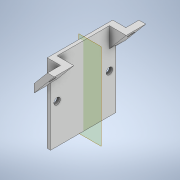
# Autodesk Inventor part: conecter bracet cover plate
Saved by Autodesk Inventor 2021 (Build 250183000, 183)
## iProperties
Created: 2022-03-10
Part Number: conecter bracet cover plate
Material: Generic
Document SubType Name: Modeling
Designer: jasmi
Density: 1 g/cm^3
Appearance: Default
Author: jasmi
Autodesk Inventor part; units mm, degrees
ref_plane "YZ Plane" through (0, 0, 0) normal (1, 0, 0) x (0, 1, 0)
ref_plane "XZ Plane" through (0, 0, 0) normal (0, 1, 0) x (-1, 0, 0)
ref_plane "XY Plane" through (0, 0, 0) normal (0, 0, 1) x (1, 0, 0)
sketch "Sketch1" plane through (0, 0, 0) normal (1, 0, 0) x (0, 1, 0)
  line L0 (76.2, 63.5) -> (0, 63.5)
  line L1 (0, 63.5) -> (0, 0)
  line L2 (0, 0) -> (76.2, 0)
  line L3 (76.2, 0) -> (76.2, 63.5)
  dimension "d0" = 76.2
  dimension "d1" = 63.5
  constraints: 8 end point, 2 parallel, 1 horizontal, 1 perpendicular
  measures "d0" distance of L1.end L2.end
  measures "d1" distance between parallel lines of L0 L2
extrude "Extrusion1" add sketch "Sketch1" along normal blind 3.175
sketch "Sketch2" plane through (3.175, 0, 0) normal (1, 0, 0) x (0, 0, -1)
  line L0 (-63.5, 76.2) -> (-63.5, 0) projected
  line L1 (0, 0) -> (0, 76.2) projected
  line L2 (0, 76.2) -> (-63.5, 76.2) projected
  point P0 (-57.15, 38.1)
  point P1 (-6.35, 38.1)
  dimension "d11" = 6.35
  dimension "d12" = 6.35
  dimension "d13" = 38.1
  dimension "d14" = 38.1
  measures "d11" distance from line of point (-57.15, 38.1) L0
  measures "d12" distance from line of point (-6.35, 38.1) L1
  measures "d13" distance from line of point (-6.35, 38.1) L2
  measures "d14" distance from line of point (-57.15, 38.1) L2
hole "Hole1" at (3.175, 38.1, 57.15) at (3.175, 38.1, 6.35) direction (-1, 0, 0) diameter 6.35 end through all
sketch "Sketch3" plane through (0, 0, 0) normal (0, 0, -1) x (-1, 0, 0)
  line L0 (-19.5018, 76.2) -> (-3.175, 56.7425)
  line L1 (-3.175, 56.7425) -> (-3.175, 76.2)
  line L2 (-3.175, 0) -> (-3.175, 76.2) projected
  line L3 (-3.175, 76.2) -> (-19.5018, 76.2)
  line L4 (0, 76.2) -> (-3.175, 76.2) projected
  point P0 (0, 0)
  dimension "d15" = 40
  dimension "d18" = 25.4
  constraints: 6 end point, 1 collinear, 1 horizontal, 1 point on line
  measures "d15" angle of L1 L0
  measures "d18" distance of L0.start L0.end
extrude "Extrusion2" add sketch "Sketch3" against normal blind 6.35
sketch "Sketch4" plane through (0, 0, 0) normal (0, 0, -1) x (-1, 0, 0)
  line L0 (0, 76.2) -> (-19.5018, 76.2) projected
  line L1 (-19.5018, 76.2) -> (0, 52.9587)
  line L2 (-19.5018, 76.2) -> (-12.8703, 76.2)
  line L3 (-12.8703, 76.2) -> (0, 60.8617)
  line L4 (-3.175, 56.7425) -> (-19.5018, 76.2) projected
  line L5 (0, 52.9587) -> (0, 60.8617)
  line L6 (0, 0) -> (0, 76.2) projected
  point P0 (-3.175, 76.2)
  dimension "d21" = 5.08
  constraints: 8 end point, 2 collinear, 1 horizontal, 1 parallel
  measures "d21" distance between parallel lines of L1 L3
extrude "Extrusion3" add sketch "Sketch4" along normal blind 12.7 contours L3 L5 L1 L0
ref_plane "Work Plane1" through (0, 0, 31.75) normal (0, 0, -1) x (-1, 0, 0)
mirror "Mirror1" about plane through (0, 0, 31.75) normal (0, 0, -1) of "Extrusion2", "Extrusion3"
sketch "Sketch5" plane through (12.8703, 76.2, -12.7) normal (-0.766, 0.6428, 0) x (0, 0, 1)
  line L0 (88.9, -20.0227) -> (88.9, 0) projected
  line L1 (76.2, -21.1374) -> (88.9, -21.1374) projected
  point P0 (12.7, -66.6455)
  point P1 (6.35, -8.4374)
  point P2 (82.55, -8.4374)
  point P3 (88.9, -15.0833)
  point P4 (88.9, -26.0768)
  dimension "d31" = 76.2
  dimension "d32" = 6.35
  dimension "d33" = 12.7
  constraints: 1 horizontal alignment
  measures "d31" distance of point (82.55, -8.437) point (6.35, -8.437)
  measures "d32" distance from line of L0 point (82.55, -8.437)
  measures "d33" distance from line of point (82.55, -8.437) L1
hole "Hole2" at (7.4469, 69.7366, -6.35) at (7.4469, 69.7366, 69.85) direction (0.766, -0.6428, 0) diameter 6.35 end through all
body "Solid1"
